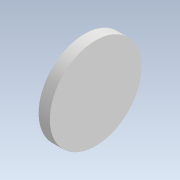
# Autodesk Inventor part: retenedor_plato
Saved by Autodesk Inventor 2021 (Build 250183000, 183)
## iProperties
Created: 2021-04-24
Part Number: retenedor_plato
Material: Genérico
Document SubType Name: Modeling
Designer: j2seb
Density: 1 g/cm^3
Appearance: Valor por defecto
Author: j2seb
Autodesk Inventor part; units mm, degrees
ref_plane "YZ Plane" through (0, 0, 0) normal (1, 0, 0) x (0, 1, 0)
ref_plane "XZ Plane" through (0, 0, 0) normal (0, 1, 0) x (-1, 0, 0)
ref_plane "XY Plane" through (0, 0, 0) normal (0, 0, 1) x (1, 0, 0)
sketch "Boceto1" plane through (0, 0, 0) normal (1, 0, 0) x (0, 1, 0)
  circle A0 centre (0, 0) radius 25
  dimension "d9" = 50
  constraints: 1 centre point, 1 coincident
  measures "d9" diameter of A0
extrude "Extrusión1" add sketch "Boceto1" along normal blind 8
sketch "Boceto2" plane through (0, 0, 0) normal (-1, 0, 0) x (0, 0, 1)
  circle A0 centre (0, 0) radius 25 projected
  constraints: 1 coincident
hole "Agujero1" at (0, 0, 0) direction (1, 0, 0) diameter 31.3762 end through all thread size "M33x1.5" class "6H" standard "ISO Metric profile"
chamfer "Chaflán1" distance 1 angle 45 4 edges at (0, -25, 0) (8, -25, 0) (0, 0, -15.6881) (8, 0, -15.6881)
sketch "Boceto3" plane through (0, 0, 0) normal (-1, 0, 0) x (0, 0, 1)
  circle A0 centre (0, 0) radius 24 projected
  circle A1 centre (0, 0) radius 25 projected
  line L0 (3, -25) -> (-3, -25)
  line L1 (-3, -25) -> (-3, -22)
  line L2 (-3, -22) -> (3, -22)
  line L3 (3, -22) -> (3, -25)
  point P0 (0, -22)
  dimension "d13" = 6
  dimension "d14" = 3
  constraints: 8 end point, 2 parallel, 1 horizontal, 1 midpoint, 1 perpendicular, 1 tangent, 1 vertical alignment
  measures "d13" distance between parallel lines of L3 L1
  measures "d14" distance between parallel lines of L2 L0
extrude "Extrusión2" cut sketch "Boceto3" against normal through all contours L1 L2 L3 A0 | A0 L3 A1 L1 | A1 L0 L1 | L3 L0 A1 picked at (-0.3341, -22.6597) picked at (0, -24.3194)
fillet "Empalme1" radius 0.5 2 edges at (4, -22, -3) (4, -22, 3)
pattern_circular "Patrón circular1" count 4 over 360 about axis through (71.1618, 0, 0) along (-1, 0, 0) of "Extrusión2", "Empalme1"
